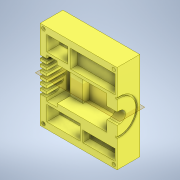
# Autodesk Inventor part: caseLowerPortionV03
Saved by Autodesk Inventor 2022.2 (Build 262287000, 287)
## iProperties
Created: 2021-08-20
Part Number: caseLowerPortionV03
Material: PC/ABS Plastic
Document SubType Name: Modeling
Designer: robst
Density: 0.357273 g/cm^3
Appearance: Smooth - Yellow
Author: robst
Autodesk Inventor part; units mm, degrees
ref_plane "YZ Plane" through (0, 0, 0) normal (1, 0, 0) x (0, 1, 0)
ref_plane "XY Plane" through (0, 0, 0) normal (0, 0, 1) x (1, 0, 0)
sketch "Sketch1" plane through (0, 0, 0) normal (0, 0, 1) x (1, 0, 0)
  line L0 (-59.35, -68.5) -> (59.35, -68.5)
  line L1 (59.35, -68.5) -> (59.35, 68.5)
  line L2 (59.35, 68.5) -> (-59.35, 68.5)
  line L3 (-59.35, 68.5) -> (-59.35, -68.5)
  line L4 (-59.35, -68.5) -> (59.35, 68.5) construction
  line L5 (59.35, -68.5) -> (-59.35, 68.5) construction
  point P0 (0, 0)
  dimension "d0" = 118.7
  dimension "d1" = 137
  constraints: 12 end point, 2 midpoint, 2 parallel, 1 horizontal, 1 perpendicular
  measures "d0" distance of L0.start L0.end
  measures "d1" distance of L1.end L0.end
extrude "MainInnerBodyExtrusion" add sketch "Sketch1" against normal blind 35
sketch "Sketch3" plane through (0, 0, 0) normal (0, 0, 1) x (1, 0, 0)
  line L0 (-13.35, -26) -> (43.65, -26)
  line L1 (43.65, -26) -> (43.65, 26)
  line L2 (43.65, 26) -> (-13.35, 26)
  line L3 (-13.35, 26) -> (-13.35, -26)
  line L4 (-13.35, -26) -> (43.65, 26) construction
  line L5 (43.65, -26) -> (-13.35, 26) construction
  line L6 (59.35, -68.5) -> (59.35, 68.5) projected
  line L7 (0, 0) -> (59.35, 0) construction
  line L8 (-59.35, -68.5) -> (-59.35, 68.5) construction
  line L9 (-59.35, 68.5) -> (-59.35, -68.5) projected
  point P0 (15.15, 0)
  point P1 (15.15, 0)
  dimension "d5" = 15.7
  dimension "d6" = 52
  dimension "d7" = 57
  constraints: 14 end point, 4 midpoint, 2 parallel, 1 horizontal, 1 perpendicular, 1 point on line
  measures "d5" distance between parallel lines of L1 L6
  measures "d6" distance of L0.end L1.end
  measures "d7" distance of L1.end L2.end
extrude "HoleForCameraCase" cut sketch "Sketch3" against normal blind 29.875
sketch "Sketch4" plane through (0, 0, 0) normal (0, 0, 1) x (1, 0, 0)
  line L0 (0, 0) -> (-59.35, 0) construction
  line L1 (-59.35, -68.5) -> (-59.35, 68.5) construction
  line L2 (-49.35, -31) -> (-33.35, -31)
  line L3 (-33.35, -31) -> (-33.35, 31)
  line L4 (-33.35, 31) -> (-49.35, 31)
  line L5 (-49.35, 31) -> (-49.35, -31)
  line L6 (-49.35, -31) -> (-33.35, 31) construction
  line L7 (-33.35, -31) -> (-49.35, 31) construction
  point P0 (-41.35, 0)
  dimension "d13" = 16
  dimension "d14" = 62
  dimension "d15" = 10
  constraints: 14 end point, 3 midpoint, 2 parallel, 1 perpendicular, 1 point on line
  measures "d13" distance of L2.start L2.end
  measures "d14" distance of L3.end L2.end
  measures "d15" distance between parallel lines of L1 L5
extrude "HoleForFan" cut sketch "Sketch4" against normal blind 31
sketch "Sketch10" plane through (0, 0, 0) normal (0, 0, 1) x (1, 0, 0)
  line L0 (-12.65, 30.5) -> (56.35, 30.5)
  line L1 (56.35, 30.5) -> (56.35, 58.5)
  line L2 (56.35, 58.5) -> (-12.65, 58.5)
  line L3 (-12.65, 58.5) -> (-12.65, 30.5)
  line L4 (-12.65, 30.5) -> (56.35, 58.5) construction
  line L5 (56.35, 30.5) -> (-12.65, 58.5) construction
  line L6 (59.35, 68.5) -> (-59.35, 68.5) projected
  line L7 (59.35, -68.5) -> (59.35, 68.5) projected
  point P0 (0, 0)
  point P1 (21.85, 44.5)
  point P2 (94.85, 8.5)
  point P3 (56.35, 44.5)
  dimension "d36" = 69
  dimension "d37" = 28
  dimension "d85" = 3
  dimension "d162" = 10
  constraints: 12 end point, 3 midpoint, 2 parallel, 1 horizontal, 1 perpendicular, 1 other
  measures "d36" distance of L1.end L2.end
  measures "d37" distance of L0.end L1.end
  measures "d162" distance between parallel lines of L2 L6
extrude "HoleForThermister" cut sketch "Sketch10" against normal blind 11
sketch "Sketch11" plane through (0, 0, 0) normal (0, 0, 1) x (1, 0, 0)
  line L0 (6.35, -58.5) -> (56.35, -58.5)
  line L1 (56.35, -58.5) -> (56.35, -41.5)
  line L2 (56.35, -41.5) -> (6.35, -41.5)
  line L3 (6.35, -41.5) -> (6.35, -58.5)
  line L4 (6.35, -58.5) -> (56.35, -41.5) construction
  line L5 (56.35, -58.5) -> (6.35, -41.5) construction
  line L6 (59.35, -68.5) -> (59.35, 68.5) projected
  line L7 (-59.35, -68.5) -> (59.35, -68.5) projected
  line L8 (43.65, -26) -> (-13.35, -26) projected
  line L9 (21.65, 64.5) -> (21.65, -64.5) projected
  point P0 (0, 0)
  point P1 (31.35, -50)
  point P2 (94.85, -8.5)
  point P3 (31.35, -41.5)
  point P4 (6.35, -50)
  point P5 (59.35, 68.5)
  dimension "d42" = 50
  dimension "d43" = 17
  dimension "d86" = 3
  dimension "d87" = 10
  constraints: 12 end point, 4 midpoint, 2 parallel, 1 horizontal, 1 perpendicular, 1 other
  measures "d42" distance of L0.start L0.end
  measures "d43" distance of L0.end L1.end
  measures "d87" distance between parallel lines of L7 L0
extrude "HoleForSensor" cut sketch "Sketch11" against normal blind 11
sketch "Sketch15" plane through (-59.35, -68.5, 0) normal (-1, 0, 0) x (0, 0, 1)
  line L0 (0, 137) -> (0, 0) projected
  line L1 (0, 137) -> (-35, 137) projected
  line L2 (-35, 0) -> (-35, 137) projected
  line L3 (0, 0) -> (-35, 0) projected
  line L4 (0, 0) -> (0, 137) projected
  line L5 (0, 94.5) -> (0, 42.5) projected
  line L6 (0, 68.5) -> (-30, 68.5) construction
  line L7 (0, 70.5) -> (-29.9333, 70.5)
  line L8 (0, 78.5) -> (-28.2843, 78.5)
  line L9 (0, 74.5) -> (-29.3939, 74.5)
  line L10 (0, 70.5) -> (0, 68.5)
  line L11 (0, 82.5) -> (-26.533, 82.5)
  line L12 (0, 86.5) -> (-24, 86.5)
  line L13 (-20.3961, 90.5) -> (0, 90.5)
  line L14 (-14.9666, 94.5) -> (0, 94.5)
  line L15 (0, 78.5) -> (0, 74.5)
  line L16 (0, 94.5) -> (0, 90.5)
  line L17 (0, 86.5) -> (0, 82.5)
  line L18 (0, 66.5) -> (-29.9333, 66.5)
  line L19 (0, 58.5) -> (-28.2843, 58.5)
  line L20 (0, 62.5) -> (-29.3939, 62.5)
  line L21 (0, 66.5) -> (0, 68.5)
  line L22 (0, 54.5) -> (-26.533, 54.5)
  line L23 (0, 50.5) -> (-24, 50.5)
  line L24 (-20.3961, 46.5) -> (0, 46.5)
  line L25 (-14.9666, 42.5) -> (0, 42.5)
  line L26 (0, 58.5) -> (0, 62.5)
  line L27 (0, 50.5) -> (0, 54.5)
  line L28 (0, 42.5) -> (0, 46.5)
  line L29 (0, 66.5) -> (0, 70.5)
  line L30 (0, 74.5) -> (0, 78.5)
  line L31 (0, 82.5) -> (0, 86.5)
  line L32 (0, 90.5) -> (0, 137)
  arc A0 (-28.2843, 78.5) -> (-29.3939, 74.5) centre (0, 68.5) ccw
  arc A1 (-14.9666, 94.5) -> (-20.3961, 90.5) centre (0, 68.5) ccw
  arc A2 (-24, 86.5) -> (-26.533, 82.5) centre (0, 68.5) ccw
  arc A3 (-29.9333, 70.5) -> (-29.9333, 66.5) centre (0, 68.5) ccw
  arc A4 (-29.3939, 62.5) -> (-28.2843, 58.5) centre (0, 68.5) ccw
  arc A5 (-26.533, 54.5) -> (-24, 50.5) centre (0, 68.5) ccw
  arc A6 (-20.3961, 46.5) -> (-14.9666, 42.5) centre (0, 68.5) ccw
  point P0 (0, 68.5)
  point P1 (0, 82)
  point P2 (0, 67.0167)
  point P3 (0, 4.25)
  point P4 (-10.198, 90.5)
  point P5 (0, 46.5)
  point P6 (0, 50.5)
  point P7 (0, 54.5)
  point P8 (0, 58.5)
  point P9 (0, 62.5)
  point P10 (0, 66.5)
  point P11 (0, 74.5)
  point P12 (0, 78.5)
  point P13 (0, 82.5)
  point P14 (0, 86.5)
  point P15 (0, 90.5)
  point P16 (0, 94.5)
  dimension "d69" = 2
  dimension "d71" = 4
  dimension "d72" = 4
  dimension "d73" = 4
  dimension "d75" = 4
  dimension "d142" = 30
  constraints: 54 end point, 15 point on circle, 15 symmetric about line, 7 centre point, 3 parallel, 3 perpendicular, 2 horizontal, 1 coincident, 1 midpoint, 1 other
  measures "d69" distance between parallel lines of L7 L6
  measures "d71" distance between parallel lines of L8 L9
  measures "d72" distance between parallel lines of L11 L8
  measures "d73" distance between parallel lines of L12 L11
  measures "d75" distance between parallel lines of L13 L14
  measures "d142" radius of A2
extrude "SlotsForRearFan" cut sketch "Sketch15" against normal up to surface (10 mm away) contours L0 L13 A1 L14 | L0 L11 A2 L12 | L25 A6 L24 L0 | L0 L9 A0 L8 | L23 A5 L22 L0 | L0 L18 A3 L7 | L19 A4 L20 L0
sketch "Sketch16" plane through (0, 0, -29.875) normal (0, 0, 1) x (1, 0, 0)
  line L0 (43.65, 26) -> (43.65, -26) projected
  line L1 (28.15, 10.765) -> (28.15, -11.235) construction
  line L2 (26.65, 10.765) -> (26.65, -11.235)
  line L3 (23.65, -11.235) -> (23.65, 10.765)
  line L4 (20.65, 8.7746) -> (20.65, -9.2446)
  line L5 (17.65, 3.5785) -> (17.65, -4.0485)
  line L6 (29.65, 10.765) -> (29.65, -11.235)
  line L7 (32.65, -11.235) -> (32.65, 10.765)
  line L8 (35.65, 8.7746) -> (35.65, -9.2446)
  line L9 (38.65, 3.5785) -> (38.65, -4.0485)
  line L10 (21.7991, 10.765) -> (23.65, 10.765)
  line L11 (23.65, -11.235) -> (21.7991, -11.235)
  line L12 (21.7991, -11.235) -> (20.65, -9.2446)
  line L13 (17.65, -4.0485) -> (15.4483, -0.235)
  line L14 (15.4483, -0.235) -> (17.65, 3.5785)
  line L15 (20.65, 8.7746) -> (21.7991, 10.765)
  line L16 (26.65, 10.765) -> (29.65, 10.765)
  line L17 (32.65, 10.765) -> (34.5009, 10.765)
  line L18 (34.5009, -11.235) -> (32.65, -11.235)
  line L19 (29.65, -11.235) -> (26.65, -11.235)
  line L20 (40.8517, -0.235) -> (38.65, -4.0485)
  line L21 (35.65, -9.2446) -> (34.5009, -11.235)
  line L22 (34.5009, 10.765) -> (35.65, 8.7746)
  line L23 (38.65, 3.5785) -> (40.8517, -0.235)
  point P0 (0, 0)
  point P1 (28.15, -0.235)
  point P2 (17.65, -0.235)
  dimension "d78" = 15.5
  dimension "d89" = 1.5
  dimension "d90" = 3
  dimension "d91" = 3
  dimension "d92" = 3
  constraints: 46 end point, 8 symmetric about line, 6 perpendicular, 3 horizontal, 3 midpoint, 2 vertical, 7 other
  measures "d78" distance from line of point (28.15, -0.235) L0
  measures "d89" distance between parallel lines of L2 L1
  measures "d90" distance between parallel lines of L3 L2
  measures "d91" distance between parallel lines of L4 L3
  measures "d92" distance from line of point (17.65, -0.235) L4
extrude "VentForCamera" cut sketch "Sketch16" against normal through all
sketch "Sketch18" plane through (59.35, -68.5, 0) normal (1, 0, 0) x (0, 0, -1)
  line L0 (0, 68.5) -> (29.6767, 68.5) construction
  arc A0 (3.875, 59.5) -> (3.875, 77.5) centre (3.875, 68.5) ccw
  line L1 (0, 0) -> (0, 137) projected
  line L2 (3.875, 77.5) -> (0, 77.5)
  line L3 (3.875, 59.5) -> (0, 59.5)
  line L4 (0, 77.5) -> (0, 59.5)
  dimension "d97" = 18
  dimension "d137" = 3.875
  constraints: 8 end point, 3 point on line, 2 perpendicular, 2 point on circle, 2 tangent, 1 centre point, 1 collinear, 1 horizontal, 1 midpoint
  measures "d97" diameter of A0
  measures "d137" distance of point (0, 68.5) A0.centre
extrude "HoleForLens" cut sketch "Sketch18" against normal blind 20
sketch "Sketch23" plane through (0, 0, 0) normal (0, 0, 1) x (1, 0, 0)
  line L0 (-54.35, -63.5) -> (54.35, -63.5) construction
  line L1 (54.35, -63.5) -> (54.35, 63.5) construction
  line L2 (54.35, 63.5) -> (-54.35, 63.5) construction
  line L3 (-54.35, 63.5) -> (-54.35, -63.5) construction
  line L4 (-54.35, -63.5) -> (54.35, 63.5) construction
  line L5 (54.35, -63.5) -> (-54.35, 63.5) construction
  line L6 (59.35, -68.5) -> (59.35, -9) projected
  line L7 (59.35, 68.5) -> (-59.35, 68.5) projected
  line L8 (-13.35, -26) -> (-13.35, 26) projected
  line L9 (-33.35, 31) -> (-33.35, -31) projected
  line L10 (-33.35, 31) -> (-33.35, -31) projected
  line L11 (-13.35, 26) -> (-33.35, 26)
  line L12 (-33.35, 26) -> (-33.35, -26)
  line L13 (-33.35, -26) -> (-13.35, -26)
  line L14 (-13.35, -26) -> (-13.35, 26)
  point P0 (0, 0)
  dimension "d106" = 5
  dimension "d108" = 5
  constraints: 20 end point, 4 coincident, 4 parallel, 2 horizontal, 2 midpoint, 2 perpendicular, 1 point on line
  measures "d106" distance between parallel lines of L1 L6
  measures "d108" distance between parallel lines of L2 L7
hole "Hole for 6-32 Insert" at (-54.35, 63.5, 0) at (54.35, 63.5, 0) at (54.35, -63.5, 0) at (-54.35, -63.5, 0) direction (0, 0, -1) diameter 4.7 depth 7.2 tip angle 118 counterbore diameter 5.54 counterbore depth 5.55
hole "Screw hole for 6-32 screw" at (-54.35, -63.5, 0) at (54.35, -63.5, 0) at (54.35, 63.5, 0) at (-54.35, 63.5, 0) direction (0, 0, -1) diameter 3.797 depth 15 tip angle 118 clearance for "Hex Machine Screw" size "#6" standard "Ansi Unified Screw Threads"
sketch "HoleFor50mmLensCover" plane through (59.35, -68.5, -35) normal (1, 0, 0) x (0, 0, -1)
  arc A0 (-31.125, 59.5) -> (-31.125, 77.5) centre (-31.125, 68.5) ccw projected
  circle A1 centre (-31.125, 69.2457) radius 27.5
  circle A2 centre (-31.125, 69.2457) radius 25
  point P0 (-35, 68.5)
  dimension "d163" = 55
  dimension "d164" = 50
  constraints: 2 centre point, 1 coincident
  measures "d163" diameter of A1
  measures "d164" diameter of A2
extrude "HoleForLensCover" cut sketch "HoleFor50mmLensCover" against normal blind 2
sketch "Sketch30" plane through (0, 0, 0) normal (0, 0, 1) x (1, 0, 0)
  line L0 (-33.35, 31) -> (-33.35, -31) projected
  line L1 (-13.35, -26) -> (-13.35, 26) projected
  line L2 (-13.35, -26) -> (-13.35, 26) projected
  line L3 (-33.35, 31) -> (-33.35, -31) projected
  line L4 (-13.35, 26) -> (-33.35, 26)
  line L5 (-33.35, 26) -> (-33.35, -26)
  line L6 (-33.35, -26) -> (-13.35, -26)
  line L7 (-13.35, -26) -> (-13.35, 26)
  line L8 (-13.35, 26) -> (43.65, 26) projected
  line L9 (43.65, -26) -> (-13.35, -26) projected
  point P0 (0, 0)
  point P1 (-33.35, -26)
  constraints: 8 end point, 2 collinear, 2 parallel, 1 horizontal, 1 perpendicular, 1 point on line
extrude "Extrusion21" cut sketch "Sketch30" against normal blind 20
sketch "Sketch31" plane through (0, 0, 0) normal (0, 0, 1) x (1, 0, 0)
  line L0 (-49.35, -58.5) -> (2.35, -58.5)
  line L1 (2.35, -58.5) -> (2.35, -35)
  line L2 (2.35, -35) -> (-49.35, -35)
  line L3 (-49.35, -35) -> (-49.35, -58.5)
  line L4 (-59.35, -26) -> (-59.35, -68.5) projected
  line L5 (-59.35, -68.5) -> (59.35, -68.5) projected
  line L6 (6.35, -58.5) -> (6.35, -41.5) projected
  line L7 (-33.35, -31) -> (-49.35, -31) projected
  line L8 (-49.35, 58.5) -> (-16.65, 58.5)
  line L9 (-16.65, 58.5) -> (-16.65, 35)
  line L10 (-16.65, 35) -> (-49.35, 35)
  line L11 (-49.35, 35) -> (-49.35, 58.5)
  line L12 (-59.35, 68.5) -> (-59.35, 26) projected
  line L13 (59.35, 68.5) -> (-59.35, 68.5) projected
  line L14 (-49.35, 31) -> (-33.35, 31) projected
  line L15 (-12.65, 30.5) -> (-12.65, 58.5) projected
  point P0 (0, 0)
  point P1 (-49.35, -46.75)
  point P2 (-41.35, -31)
  point P3 (-33, 58.5)
  dimension "d169" = 10
  dimension "d170" = 10
  dimension "d171" = 4
  dimension "d172" = 4
  dimension "d173" = 10
  dimension "d174" = 10
  dimension "d175" = 4
  dimension "d176" = 4
  constraints: 16 end point, 4 parallel, 3 midpoint, 2 horizontal, 2 perpendicular
  measures "d169" distance from line of point (-49.35, -46.75) L4
  measures "d170" distance between parallel lines of L5 L0
  measures "d171" distance between parallel lines of L1 L6
  measures "d172" distance from line of L2 point (-41.35, -31)
  measures "d173" distance between parallel lines of L12 L11
  measures "d174" distance from line of point (-33, 58.5) L13
  measures "d175" distance between parallel lines of L14 L10
  measures "d176" distance between parallel lines of L15 L9
extrude "Extrusion22" cut sketch "Sketch31" against normal blind 20
equation "\"d0\" = caseLength"
equation "\"d2\" = caseDepth"
equation "\"d5\" = lensLength"
equation "\"d6\" = cameraWidth"
equation "\"d7\" = cameraLength"
equation "\"d13\" = fanDepth"
equation "\"d14\" = fanWidth"
equation "\"d15\" = rearWallThickness"
equation "\"d36\" = thermisterLength"
equation "\"d37\" = thermisterWidth"
equation "\"d85\" = frontWallThickness"
equation "\"d42\" = sensorLength"
equation "\"d43\" = sensorWidth"
equation "\"d86\" = frontWallThickness"
equation "\"d87\" = outsideWallThickness"
equation "\"outsideWallThickness\" = 10"
equation "\"caseWidth\" = 137"
equation "\"lensLength\" = 15.7"
equation "\"lensDiameter\" = 17"
equation "\"thickenDistance\" = 1"
equation "\"bottomOfCaseWallThickness\" = 3"
equation "\"rearWallThickness\" = 10"
equation "\"maxComponentDepth\" = 32"
equation "\"caseDepth\" = maxComponentDepth + bottomOfCaseWallThickness"
equation "\"fanCutoutDepth\" = 0.5 * fanLength + extraCutoutDepth + thickenDistance"
equation "\"caseLength\" = 118.7"
equation "\"frontWallThickness\" = 3"
equation "\"d95\" = lensDiameter"
equation "\"extraCutoutDepth\" = 15.5"
equation "\"halfFanDepth\" = 31"
equation "\"cameraCaseDepth\" = 57.75"
equation "\"halfCameraCaseDepth\" = 29.875"
equation "\"halfThirmesterDepth\" = 11"
equation "\"halfSensorDepth\" = 11"
equation "\"depthForLensSlot\" = 3.875"
equation "\"cameraWidth\" = 52"
equation "\"cameraLength\" = 57"
equation "\"fanDepth\" = 16"
equation "\"fanWidth\" = 62"
equation "\"thermisterLength\" = 69"
equation "\"thermisterWidth\" = 28"
equation "\"sensorLength\" = 50"
equation "\"sensorWidth\" = 17"
equation "\"fanLength\" = 60"
body "Solid1"
